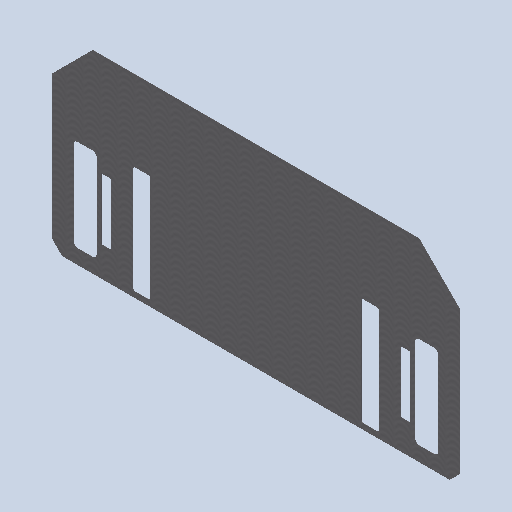
# Autodesk Inventor part: PlanchaBaseInferior
Saved by Autodesk Inventor 2022.1 (Build 261234000, 234)
## iProperties
Created: 2021-09-22
Part Number: PlanchaBaseInferior
Material: Steel, Mild, Welded
Document SubType Name: Sheet Metal
Designer: Andres
Density: 7.85 g/cm^3
Sheet Metal Rule: Por defecto_mm
Appearance: Weld - Steel Mild
Author: Andres
Autodesk Inventor part; units mm, degrees
ref_plane "YZ Plane" through (0, 0, 0) normal (1, 0, 0) x (0, 1, 0)
ref_plane "XZ Plane" through (0, 0, 0) normal (0, 1, 0) x (-1, 0, 0)
ref_plane "XY Plane" through (0, 0, 0) normal (0, 0, 1) x (1, 0, 0)
sketch "Sketch1" plane through (0, 0, 0) normal (0, 0, 1) x (1, 0, 0)
  line L0 (125.9853, -345.9853) -> (-56.337, -345.9853)
  line L1 (-56.337, -345.9853) -> (-69.0147, -333.3076)
  line L2 (-69.0147, -333.3076) -> (-69.0147, 16.337)
  line L3 (-69.0147, 16.337) -> (23.663, 109.0147)
  line L4 (23.663, 109.0147) -> (125.9853, 109.0147)
  line L5 (750.9853, 109.0147) -> (853.3076, 109.0147)
  line L6 (570.9853, 109.0147) -> (725.9853, 109.0147)
  line L7 (150.9853, 109.0147) -> (305.9853, 109.0147)
  line L8 (330.9853, 109.0147) -> (545.9853, 109.0147)
  line L9 (853.3076, 109.0147) -> (945.9853, 16.337)
  line L10 (945.9853, 16.337) -> (945.9853, -333.3076)
  line L11 (945.9853, -333.3076) -> (933.3076, -345.9853)
  line L12 (933.3076, -345.9853) -> (750.9853, -345.9853)
  line L13 (943.663, -370.9853) -> (750.9853, -370.9853)
  line L14 (970.9853, -343.663) -> (943.663, -370.9853)
  line L15 (970.9853, 26.6924) -> (970.9853, -343.663)
  line L16 (863.663, 134.0147) -> (970.9853, 26.6924)
  line L17 (13.3076, 134.0147) -> (863.663, 134.0147)
  line L18 (-94.0147, 26.6924) -> (13.3076, 134.0147)
  line L19 (-94.0147, -343.663) -> (-94.0147, 26.6924)
  line L20 (-66.6924, -370.9853) -> (-94.0147, -343.663)
  line L21 (125.9853, -370.9853) -> (-66.6924, -370.9853)
  line L22 (750.9853, -370.9853) -> (125.9853, -370.9853)
  line L23 (125.9853, -370.9853) -> (125.9853, -345.9853)
  line L24 (125.9853, 109.0147) -> (125.9853, 121.5147)
  line L25 (125.9853, 121.5147) -> (150.9853, 121.5147)
  line L26 (150.9853, 109.0147) -> (150.9853, 121.5147)
  line L27 (305.9853, 121.5147) -> (305.9853, 109.0147)
  line L28 (305.9853, 121.5147) -> (330.9853, 121.5147)
  line L29 (330.9853, 121.5147) -> (330.9853, 109.0147)
  line L30 (545.9853, 121.5147) -> (545.9853, 109.0147)
  line L31 (545.9853, 121.5147) -> (570.9853, 121.5147)
  line L32 (570.9853, 121.5147) -> (570.9853, 109.0147)
  line L33 (725.9853, 109.0147) -> (725.9853, 121.5147)
  line L34 (725.9853, 121.5147) -> (750.9853, 121.5147)
  line L35 (750.9853, 109.0147) -> (750.9853, 121.5147)
  line L36 (750.9853, -370.9853) -> (750.9853, -345.9853)
extrude "Plate1" add sketch "Sketch1" along normal blind 0.5
sketch "Sketch2" plane through (0, 0, 0.5) normal (0, 0, 1) x (1, 0, 0)
  line L0 (943.663, -370.9853) -> (-66.6924, -370.9853) projected
  line L1 (970.9853, -343.663) -> (943.663, -370.9853) projected
  line L2 (970.9853, 26.6924) -> (970.9853, -343.663) projected
  line L3 (863.663, 134.0147) -> (970.9853, 26.6924) projected
  line L4 (13.3076, 134.0147) -> (863.663, 134.0147) projected
  line L5 (-94.0147, 26.6924) -> (13.3076, 134.0147) projected
  line L6 (-94.0147, -343.663) -> (-94.0147, 26.6924) projected
  line L7 (-66.6924, -370.9853) -> (-94.0147, -343.663) projected
  line L8 (35.9853, 91.5147) -> (35.9853, -358.4853) projected
  line L9 (60.9853, 91.5147) -> (60.9853, -358.4853) projected
  line L10 (815.9853, 121.5147) -> (815.9853, -358.4853) projected
  line L11 (840.9853, 121.5147) -> (840.9853, -358.4853) projected
  line L12 (-31.5147, -323.1151) -> (-31.5147, -103.1151) projected
  line L13 (18.4853, -103.1151) -> (18.4853, -323.1151) projected
  line L14 (858.0889, -323.1151) -> (858.0889, -103.1151) projected
  line L15 (908.0889, -103.1151) -> (908.0889, -323.1151) projected
  line L16 (-26.5147, -98.1151) -> (13.4853, -98.1151)
  arc A0 (-26.5147, -98.1151) -> (-31.5147, -103.1151) centre (-26.5147, -103.1151) ccw
  arc A1 (18.4853, -103.1151) -> (13.4853, -98.1151) centre (13.4853, -103.1151) ccw
  line L17 (-26.5147, -328.1151) -> (13.4853, -328.1151)
  arc A2 (13.4853, -328.1151) -> (18.4853, -323.1151) centre (13.4853, -323.1151) ccw
  arc A3 (-31.5147, -323.1151) -> (-26.5147, -328.1151) centre (-26.5147, -323.1151) ccw
  arc A4 (903.0889, -328.1151) -> (908.0889, -323.1151) centre (903.0889, -323.1151) ccw
  line L18 (903.0889, -328.1151) -> (863.0889, -328.1151)
  arc A5 (858.0889, -323.1151) -> (863.0889, -328.1151) centre (863.0889, -323.1151) ccw
  arc A6 (908.0889, -103.1151) -> (903.0889, -98.1151) centre (903.0889, -103.1151) ccw
  arc A7 (863.0889, -98.1151) -> (858.0889, -103.1151) centre (863.0889, -103.1151) ccw
  line L19 (903.0889, -98.1151) -> (863.0889, -98.1151)
  line L20 (23.4853, -323.1151) -> (23.4853, -103.1151)
  arc A8 (23.4853, -103.1151) -> (13.4853, -93.1151) centre (13.4853, -103.1151) ccw
  line L21 (13.4853, -93.1151) -> (-26.5147, -93.1151)
  arc A9 (-26.5147, -93.1151) -> (-36.5147, -103.1151) centre (-26.5147, -103.1151) ccw
  line L22 (-36.5147, -103.1151) -> (-36.5147, -323.1151)
  arc A10 (-36.5147, -323.1151) -> (-26.5147, -333.1151) centre (-26.5147, -323.1151) ccw
  line L23 (-26.5147, -333.1151) -> (13.4853, -333.1151)
  arc A11 (13.4853, -333.1151) -> (23.4853, -323.1151) centre (13.4853, -323.1151) ccw
  line L24 (913.0889, -323.1151) -> (913.0889, -103.1151)
  arc A12 (913.0889, -103.1151) -> (903.0889, -93.1151) centre (903.0889, -103.1151) ccw
  line L25 (903.0889, -93.1151) -> (863.0889, -93.1151)
  arc A13 (863.0889, -93.1151) -> (853.0889, -103.1151) centre (863.0889, -103.1151) ccw
  line L26 (853.0889, -103.1151) -> (853.0889, -323.1151)
  arc A14 (853.0889, -323.1151) -> (863.0889, -333.1151) centre (863.0889, -323.1151) ccw
  line L27 (863.0889, -333.1151) -> (903.0889, -333.1151)
  arc A15 (903.0889, -333.1151) -> (913.0889, -323.1151) centre (903.0889, -323.1151) ccw
  line L28 (35.9853, -293.1151) -> (60.9853, -293.1151)
  line L29 (35.9853, -133.1151) -> (60.9853, -133.1151)
  line L30 (840.9853, -133.1151) -> (815.9853, -133.1151)
  line L31 (815.9853, -293.1151) -> (840.9853, -293.1151)
  point P0 (438.4853, 79.5147)
  dimension "d9" = 45
  dimension "d19" = 5
  dimension "d20" = 5
  dimension "d21" = 40
  dimension "d22" = 40
  dimension "d23" = 40
  dimension "d24" = 40
  constraints: 32 end point, 32 point on circle, 16 centre point, 8 point on line, 5 horizontal, 3 perpendicular, 38 other
  measures "d19" distance between parallel lines of L13 L20
  measures "d20" distance between parallel lines of L15 L24
  measures "d21" distance between parallel lines of L23 L28
  measures "d22" distance between parallel lines of L21 L29
  measures "d23" distance between parallel lines of L25 L30
  measures "d24" distance between parallel lines of L31 L27
extrude "Cut1" cut sketch "Sketch2" against normal through all contours L29 L9 L28 L8 | L30 L11 L31 L10 | L12 A0 L16 A1 L13 A2 L17 A3 | L14 A7 L19 A6 L15 A4 L18 A5 | A11 L23 A10 L22 A9 L21 A8 L20 | A15 L27 A14 L26 A13 L25 A12 L24
sketch "Boceto3" plane through (0, 0, 0.5) normal (0, 0, 1) x (1, 0, 0)
  line L0 (123.4853, -355.9853) -> (158.4853, -355.9853)
  line L1 (163.4853, -350.9853) -> (163.4853, -80.9853)
  line L2 (158.4853, -75.9853) -> (123.4853, -75.9853)
  line L3 (118.4853, -80.9853) -> (118.4853, -350.9853)
  line L4 (78.4853, -31.4853) -> (78.4853, -319.4853) projected
  line L5 (438.4853, 103.5147) -> (438.4853, -370.4853)
  line L6 (753.4853, -355.9853) -> (718.4853, -355.9853)
  line L7 (713.4853, -350.9853) -> (713.4853, -80.9853)
  line L8 (718.4853, -75.9853) -> (753.4853, -75.9853)
  line L9 (758.4853, -80.9853) -> (758.4853, -350.9853)
  arc A0 (158.4853, -355.9853) -> (163.4853, -350.9853) centre (158.4853, -350.9853) ccw
  arc A1 (118.4853, -350.9853) -> (123.4853, -355.9853) centre (123.4853, -350.9853) ccw
  arc A2 (123.4853, -75.9853) -> (118.4853, -80.9853) centre (123.4853, -80.9853) ccw
  arc A3 (163.4853, -80.9853) -> (158.4853, -75.9853) centre (158.4853, -80.9853) ccw
  arc A4 (758.4853, -80.9853) -> (753.4853, -75.9853) centre (753.4853, -80.9853) ccw
  arc A5 (718.4853, -75.9853) -> (713.4853, -80.9853) centre (718.4853, -80.9853) ccw
  arc A6 (713.4853, -350.9853) -> (718.4853, -355.9853) centre (718.4853, -350.9853) ccw
  arc A7 (753.4853, -355.9853) -> (758.4853, -350.9853) centre (753.4853, -350.9853) ccw
  line L10 (943.663, -370.9853) -> (-66.6924, -370.9853) projected
  point P0 (0, 0)
  point P1 (118.4853, -355.9853)
  point P2 (163.4853, -355.9853)
  point P3 (163.4853, -75.9853)
  point P4 (118.4853, -75.9853)
  point P5 (758.4853, -355.9853)
  point P6 (713.4853, -355.9853)
  point P7 (713.4853, -75.9853)
  point P8 (758.4853, -75.9853)
  dimension "d9" = 45
  dimension "d10" = 280
  dimension "d13" = 5
  dimension "d16" = 275
  dimension "d17" = 15
  constraints: 18 end point, 16 point on circle, 16 point on line, 16 tangent, 8 centre point, 7 equal radius, 4 symmetric about line, 3 perpendicular, 1 horizontal
  measures "d9" distance of point (163.485, -75.985) point (118.485, -75.985)
  measures "d10" distance of point (163.485, -355.985) point (163.485, -75.985)
  measures "d13" radius of A0
  measures "d16" distance between parallel lines of L5 L1
  measures "d17" distance between parallel lines of L10 L0
extrude "Cortar2" cut sketch "Boceto3" against normal blind 0.5
equation "\"d6\" = Thickness"
equation "\"d14\" = Thickness"
equation "\"d0\" = Thickness"
equation "\"BendRadius\" = Thickness"
equation "\"BendReliefWidth\" = Thickness"
equation "\"BendReliefDepth\" = 0.5 * Thickness"
equation "\"CornerReliefSize\" = 4 * Thickness"
equation "\"MinimumRemnant\" = 2 * Thickness"
equation "\"TransitionRadius\" = BendRadius"
equation "\"JacobiRadiusSize\" = BendRadius"
equation "\"GapSize\" = Thickness"
equation "\"Thickness\" = 0.5"
body "Solid1"
